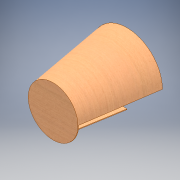
# Autodesk Inventor part: Topf
Saved by Autodesk Inventor 2017.3 (Build 213257000, 257)
## iProperties
Created: 2020-01-20
Part Number: Topf
Material: Concrete
Document SubType Name: Modeling
Designer: Ole Simmering
Density: 2.40731 g/cm^3
Appearance: Cherry - Natural Low Gloss
Author: Ole Simmering
Autodesk Inventor part; units mm, degrees
ref_plane "YZ Plane" through (0, 0, 0) normal (1, 0, 0) x (0, 1, 0)
ref_plane "XY Plane" through (0, 0, 0) normal (0, 0, 1) x (1, 0, 0)
sketch "Sketch1" plane through (0, 0, 0) normal (0, 1, 0) x (-1, 0, 0)
  circle A0 centre (0, 0) radius 87.5
  dimension "d0" = 175
  constraints: 1 centre point, 1 coincident
  measures "d0" diameter of A0
ref_plane "Work Plane1" through (0, 260, 0) normal (0, 1, 0) x (-1, 0, 0)
sketch "Sketch2" plane through (0, 260, 0) normal (0, 1, 0) x (-1, 0, 0)
  circle A0 centre (0, 0) radius 125
  dimension "d2" = 250
  constraints: 1 centre point, 1 coincident
  measures "d2" diameter of A0
loft "Loft1" add profiles "Sketch1", "Sketch2"
shell "Shell1" thickness 2.5 removed faces 1 at (0.6944, 260, 22.8612)
sketch "Sketch3" plane through (0, 260, 0) normal (0, 1, 0) x (1, 0, 0)
  line L0 (0, 0) -> (156, 0)
  line L1 (0, 0) -> (0, 209)
  line L2 (0, 209) -> (156, 209)
  line L3 (156, 209) -> (156, 0)
  constraints: 8 end point, 2 horizontal, 2 vertical
extrude "Extrusion1" cut sketch "Sketch3" against normal up to surface (257.5 mm away)
body "Solid1"
